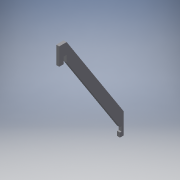
# Autodesk Inventor part: TrayPanelK
Saved by Autodesk Inventor 2017 (Build 210142000, 142)
## iProperties
Created: 2019-06-27
Part Number: TrayPanelK
Material: Generic
Document SubType Name: Modeling
Designer: DDeGo
Density: 1 g/cm^3
Appearance: Default
Author: DDeGo
Autodesk Inventor part; units mm, degrees
ref_plane "YZ Plane" through (0, 0, 0) normal (1, 0, 0) x (0, 1, 0)
ref_plane "XZ Plane" through (0, 0, 0) normal (0, 1, 0) x (-1, 0, 0)
ref_plane "XY Plane" through (0, 0, 0) normal (0, 0, 1) x (1, 0, 0)
sketch "Sketch1" plane through (0, 0, 0) normal (1, 0, 0) x (0, 1, 0)
  point P0 (0, 0)
sketch "Sketch2" plane through (0, 0, 0) normal (1, 0, 0) x (0, 1, 0)
  line L0 (2.75, 0) -> (50.125, -75)
  line L1 (50.125, -75) -> (51.625, -75)
  line L2 (51.625, -75) -> (51.625, -79.2)
  line L3 (51.625, -79.2) -> (50.125, -79.2)
  line L4 (50.125, -79.2) -> (50.125, -83.2)
  line L5 (50.125, -83.2) -> (54.625, -83.2)
  line L6 (54.625, -83.2) -> (54.625, -66.124)
  line L7 (54.625, -66.124) -> (2.75, 16)
  line L8 (2.75, 16) -> (0, 16)
  line L9 (0, 0) -> (0, 6)
  line L10 (0, 6) -> (2.75, 6)
  line L11 (2.75, 6) -> (2.75, 0)
  line L12 (0, 0) -> (2.75, 0) construction
  line L13 (50.125, -75) -> (50.125, -79.2) construction
  line L14 (0, 6) -> (0, 16) construction
  line L15 (2.75, 6) -> (2.75, 16) construction
  line L16 (0, 0) -> (-4, 0)
  line L17 (-4, 0) -> (-4, 16)
  line L18 (-4, 16) -> (0, 16)
  point P0 (0, 0)
  dimension "d37" = 2.75
  dimension "d40" = 6
  dimension "d42" = 1.5
  dimension "d43" = 3
  dimension "d44" = 4
  dimension "d45" = 10
  dimension "d60" = 4.2
  dimension "d61" = 81
  dimension "d62" = 4
  dimension "d64" = 48.875
  constraints: 38 end point, 8 perpendicular, 4 horizontal, 4 vertical, 2 parallel, 1 coincident
  measures "d37" distance between parallel lines of L11 L9
  measures "d40" distance of L10.end L0.start
  measures "d42" distance between parallel lines of L4 L2
  measures "d43" distance between parallel lines of L6 L2
  measures "d44" distance between parallel lines of L5 L3
  measures "d45" distance between parallel lines of L8 L10
  measures "d60" distance between parallel lines of L3 L1
  measures "d61" distance between parallel lines of L1 L10
  measures "d62" distance of L9.start L16.end
  measures "d64" distance between parallel lines of L11 L2
extrude "Extrusion1" add sketch "Sketch2" along normal blind 2.75
body "Solid1"
